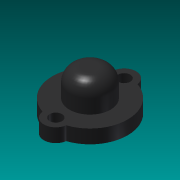
# Autodesk Inventor part: candynamix_mini_ballcaster
Saved by Autodesk Inventor 2015 (Build 190159000, 159)
## iProperties
Created: 2018-12-02
Part Number: candynamix_mini_ballcaster
Material: Generic
Document SubType Name: Modeling
Designer: tlsru
Density: 1 g/cm^3
Appearance: 고무 - 검은색
Author: tlsru
Autodesk Inventor part; units mm, degrees
ref_plane "YZ Plane" through (0, 0, 0) normal (1, 0, 0) x (0, 1, 0)
ref_plane "XZ Plane" through (0, 0, 0) normal (0, 1, 0) x (-1, 0, 0)
ref_plane "XY Plane" through (0, 0, 0) normal (0, 0, 1) x (1, 0, 0)
sketch "스케치1" plane through (0, 0, 0) normal (0, 0, 1) x (1, 0, 0)
  line L0 (-24.8745, -28.5) -> (-24.8745, -22.5) projected
  line L1 (-24.8745, -22.5) -> (-24.6915, -22.5) projected
  line L2 (4.8745, -22.5) -> (4.8745, -28.5) projected
  line L3 (30, -28.5) -> (4.8745, -28.5) projected
  line L4 (30, 27.5) -> (30, -28.5) projected
  line L5 (30, 27.5) -> (4.8745, 27.5) projected
  line L6 (4.8745, 27.5) -> (4.8745, 21.5) projected
  line L7 (-24.6915, 21.5) -> (-24.8745, 21.5) projected
  line L8 (-24.8745, 21.5) -> (-24.8745, 27.5) projected
  line L9 (17, -7.5) -> (25, -7.5)
  line L10 (25, -7.5) -> (25, 6.5)
  line L11 (25, 6.5) -> (17, 6.5)
  line L12 (17, 6.5) -> (17, -7.5)
  arc A0 (19.7598, -5.3438) -> (22.2402, -5.3438) centre (21, -5.5) ccw
  arc A1 (22.2402, 4.3437) -> (19.7598, 4.3437) centre (21, 4.5) ccw
  circle A2 centre (21, -5.5) radius 0.9
  circle A3 centre (21, 4.5) radius 0.9
  arc A4 (19.7598, 4.3437) -> (19.7598, -5.3438) centre (21, -0.5) ccw
  arc A5 (22.2402, -5.3438) -> (22.2402, 4.3437) centre (21, -0.5) ccw
  circle A6 centre (21, -5.5) radius 0.9 projected
  circle A7 centre (21, 4.5) radius 0.9 projected
  line L13 (-21.6915, -12.5) -> (-21.6915, 11.5) projected
  line L14 (4, 11.5) -> (4, -12.5) projected
  line L15 (-24.8745, 27.5) -> (-33, 27.5) projected
  line L16 (-33, -28.5) -> (-33, 27.5) projected
  line L17 (-24.8745, -28.5) -> (-33, -28.5) projected
  line L18 (7, -22.5) -> (4.8745, -22.5) projected
  line L19 (4.8745, 21.5) -> (7, 21.5) projected
  line L20 (7, 21.5) -> (7, 20) projected
  line L21 (7, 20) -> (-24.6915, 20) projected
  line L22 (-24.6915, 20) -> (-24.6915, 21.5) projected
  line L23 (-24.6915, -22.5) -> (-24.6915, -21) projected
  line L24 (-24.6915, -21) -> (7, -21) projected
  line L25 (7, -21) -> (7, -22.5) projected
  line L26 (4, -12.5) -> (-21.6915, -12.5) projected
  line L27 (-21.6915, 11.5) -> (4, 11.5) projected
  point P0 (0, 0)
  dimension "d0" = 8
  dimension "d1" = 5
  dimension "d2" = 14
  dimension "d3" = 56
  dimension "d4" = 21
  dimension "d5" = 2.5
  dimension "d6" = 2.5
  dimension "d7" = 10
  dimension "d8" = 2
  dimension "d9" = 4
  dimension "d10" = 4
  dimension "d11" = 1.8
  dimension "d12" = 1.8
  dimension "d13" = 21
  dimension "d14" = 2
  constraints: 8 end point, 8 point on circle, 6 centre point, 2 coincident, 2 parallel, 1 horizontal, 1 perpendicular
  measures "d0" distance between parallel lines of L12 L10
  measures "d1" distance between parallel lines of L4 L10
  measures "d2" distance of L11.end L9.start
  measures "d3" distance of L4.start L3.start
  measures "d4" distance between parallel lines of L5 L11
  measures "d5" diameter of A0
  measures "d6" diameter of A1
  measures "d7" distance of A1.centre A0.centre
  measures "d8" distance from line of L11 A1.centre
  measures "d9" distance from line of L12 A0.centre
  measures "d10" distance from line of L12 A1.centre
  measures "d11" diameter of A2
  measures "d12" diameter of A3
  measures "d13" distance between parallel lines of L3 L9
  measures "d14" distance from line of L9 A0.centre
extrude "돌출1" add sketch "스케치1" along normal blind 1 contours A4 L12 | L12 A4 A1 A5 L10 A0 | L10 A5
sketch "스케치2" plane through (0, 0, 1) normal (0, 0, 1) x (1, 0, 0)
  arc A0 (19.7598, 4.3437) -> (19.7598, -5.3438) centre (21, -0.5) ccw projected
  arc A1 (22.2402, 4.3437) -> (19.7598, 4.3437) centre (21, 4.5) ccw projected
  arc A2 (22.2402, -5.3438) -> (22.2402, 4.3437) centre (21, -0.5) ccw projected
  arc A3 (19.7598, -5.3438) -> (22.2402, -5.3438) centre (21, -5.5) ccw projected
  arc A4 (19.2637, 4.7187) -> (19.2637, -5.7188) centre (21, -0.5) ccw
  arc A5 (22.7363, 4.7187) -> (19.2637, 4.7187) centre (21, 4.5) ccw
  arc A6 (22.7363, -5.7188) -> (22.7363, 4.7187) centre (21, -0.5) ccw
  arc A7 (19.2637, -5.7188) -> (22.7363, -5.7188) centre (21, -5.5) ccw
  point P0 (0, 0)
  dimension "d17" = 0.5
  constraints: 8 point on circle, 4 centre point, 3 other
  measures "d17" radial gap between concentric circles of A0 A4
extrude "돌출2" add sketch "스케치2" against normal blind 1
sketch "스케치3" plane through (0, 0, 1) normal (0, 0, 1) x (1, 0, 0)
  arc A0 (19.2637, 4.7187) -> (19.2637, -5.7188) centre (21, -0.5) ccw projected
  arc A1 (19.2637, -5.7188) -> (22.7363, -5.7188) centre (21, -5.5) ccw projected
  arc A2 (22.7363, -5.7188) -> (22.7363, 4.7187) centre (21, -0.5) ccw projected
  arc A3 (22.7363, 4.7187) -> (19.2637, 4.7187) centre (21, 4.5) ccw projected
  circle A4 centre (21, 4.5) radius 0.9 projected
  circle A5 centre (21, -5.5) radius 0.9 projected
  point P0 (0, 0)
extrude "돌출3" add sketch "스케치3" along normal blind 1
sketch "스케치4" plane through (0, 0, 2) normal (0, 0, 1) x (1, 0, 0)
  circle A0 centre (21, -5.5) radius 0.9 projected
  circle A1 centre (21, 4.5) radius 0.9 projected
  arc A2 (19.2637, 4.7187) -> (19.2637, -5.7188) centre (21, -0.5) ccw projected
  arc A3 (19.2637, -5.7188) -> (22.7363, -5.7188) centre (21, -5.5) ccw projected
  arc A4 (22.7363, -5.7188) -> (22.7363, 4.7187) centre (21, -0.5) ccw projected
  arc A5 (22.7363, 4.7187) -> (19.2637, 4.7187) centre (21, 4.5) ccw projected
  circle A6 centre (21, -0.5) radius 3
  point P0 (0, 0)
  dimension "d22" = 6
  constraints: 1 centre point, 1 coincident
  measures "d22" diameter of A6
extrude "돌출4" add sketch "스케치4" along normal blind 4 contours A6
fillet "모깎기1" radius 2 1 edges at (18, -0.5, 6)
